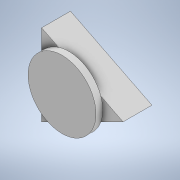
# Autodesk Inventor part: OkBtn
Saved by Autodesk Inventor 2020.1 (Build 241239000, 239)
## iProperties
Created: 2019-09-04
Part Number: OkBtn
Material: Generic
Document SubType Name: Modeling
Designer: matteo.spadetto-1
Density: 1 g/cm^3
Appearance: Default
Author: matteo.spadetto-1
Autodesk Inventor part; units mm, degrees
ref_plane "YZ Plane" through (0, 0, 0) normal (1, 0, 0) x (0, 1, 0)
ref_plane "XZ Plane" through (0, 0, 0) normal (0, 1, 0) x (-1, 0, 0)
ref_plane "XY Plane" through (0, 0, 0) normal (0, 0, 1) x (1, 0, 0)
sketch "Sketch1" plane through (0, 0, 0) normal (0, 0, 1) x (1, 0, 0)
  line L0 (0, 12) -> (0, 0)
  line L1 (0, 0) -> (12, 6)
  line L2 (12, 6) -> (0, 12)
  constraints: 6 end point
extrude "Extrusion1" add sketch "Sketch1" along normal blind 4.25
sketch "Sketch2" plane through (0, 0, 4.25) normal (0, 0, 1) x (1, 0, 0)
  line L0 (0, 0) -> (12, 6) projected
  line L1 (0, 12) -> (0, 0) projected
  line L2 (12, 6) -> (0, 12) projected
  line L3 (0, 6) -> (8, 6)
  line L4 (4, 4) -> (4, 8)
  circle A0 centre (4, 6) radius 5
  dimension "d7" = 10
  constraints: 4 end point, 2 midpoint, 1 centre point, 1 horizontal, 1 vertical
  measures "d7" diameter of A0
extrude "Extrusion3" add sketch "Sketch2" along normal blind 1 contours A0 L1 L2 L0 | L0 A0 | A0 L1 | A0 L2
body "Solid1"
